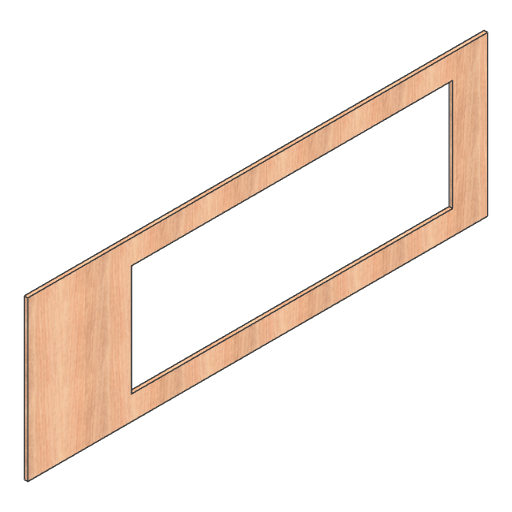
# Autodesk Inventor part: CUT PART G-01
Saved by Autodesk Inventor 2023.2 (Build 272271000, 271)
## iProperties
Created: 2022-11-02
Part Number: CUT PART G-01
Material: Wood (Birch)
Document SubType Name: Modeling
Designer: GUT
Density: 0.55 g/cm^3
Appearance: Birch - Natural Polished
Mass: 2906.48 g
Surface Area: 9671.5 cm^2
Volume: 5284.5 cm^3
b: 545,000 mm
d1: 1575,000 mm
d2: 12,000 mm
d3: 0,00 deg
d4: 380,000 mm
d5: 82,500 mm
d6: 1100,000 mm
d8: 120,000 mm
d10: 0,00 deg
Author: GUT
Autodesk Inventor part; units mm, degrees
ref_plane "YZ Plane" through (0, 0, 0) normal (1, 0, 0) x (0, 1, 0)
ref_plane "XZ Plane" through (0, 0, 0) normal (0, 1, 0) x (-1, 0, 0)
ref_plane "XY Plane" through (0, 0, 0) normal (0, 0, 1) x (1, 0, 0)
sketch "Sketch1" plane through (0, 0, 0) normal (1, 0, 0) x (0, 1, 0)
  line L0 (130.7193, 523.9242) -> (675.7193, 523.9242)
  line L1 (675.7193, 523.9242) -> (675.7193, -1051.0758)
  line L2 (675.7193, -1051.0758) -> (130.7193, -1051.0758)
  line L3 (130.7193, -1051.0758) -> (130.7193, 523.9242)
  line L4 (213.2193, -931.0758) -> (593.2193, -931.0758)
  line L5 (593.2193, -931.0758) -> (593.2193, 168.9242)
  line L6 (593.2193, 168.9242) -> (213.2193, 168.9242)
  line L7 (213.2193, 168.9242) -> (213.2193, -931.0758)
  point P0 (0, 0)
  dimension "b" = 545
  dimension "d1" = 1575
  dimension "d4" = 380
  dimension "d5" = 82.5
  dimension "d6" = 1100
  dimension "d8" = 120
  constraints: 16 end point, 4 parallel, 2 horizontal, 2 perpendicular
  measures "b" distance of L1.end L2.end
  measures "d1" distance of L0.end L1.end
  measures "d4" distance of L5.end L6.end
  measures "d5" distance between parallel lines of L1 L5
  measures "d6" distance of L4.end L5.end
  measures "d8" distance between parallel lines of L2 L4
extrude "Extrusion1" add sketch "Sketch1" along normal blind 12 contours L0 L1 L2 L3 | L7 L6 L5 L4
extrude "Extrusion2" cut sketch "Sketch1" along normal up to next contours L7 L6 L5 L4
equation "\"d5\" = -0.5 * d4 + 0.5 * b"
body "Solid1"
